Autodesk Fusion 360 part; units mm, degrees
(part 2 of 2)
sketch "Skizze22" plane through (0, -5, 0) normal (0, -1, 0) x (1, 0, 0)
  line L0 (186.6306, 4.2829) -> (187.8211, 23.7465)
  line L1 (187.8211, 23.7465) -> (186.6306, 24.2829)
  line L2 (186.6306, 24.2829) -> (151.6306, 24.2829)
  line L3 (151.6306, 24.2829) -> (151.6306, 40.8836)
  line L4 (-70, 29.3498) -> (-70, 5)
  line L5 (-70, 5) -> (0, 5)
  line L6 (0, 5) -> (0, 4)
  line L7 (0, 4) -> (20, 4)
  line L8 (20, 4) -> (20, 5)
  line L9 (20, 5) -> (149.0505, 5)
  line L10 (87.5, 37.1956) -> (87.5, 52.1956)
  arc A0 (87.5, 52.1956) -> (72.5, 52.1956) centre (80, 52.1956) ccw
  line L11 (72.5, 52.1956) -> (72.5, 37.1956)
  arc A1 (72.5, 37.1956) -> (87.5, 37.1956) centre (80, 37.1956) ccw
  line L12 (80, 37.1956) -> (80, 52.1956) construction
  spline S0 degree 3 poles (14.5724, 48.6404) (30.2605, 50.3322) (46.1682, 51.5352) (61.9632, 52) knots -4.74056 -4.74056 -4.74056 -4.74056 0 0 0 0
  line L13 (151.6306, 4.2829) -> (186.6306, 4.2829)
  arc A2 (151.6306, 4.2829) -> (149.0505, 5) centre (149.0505, 0) ccw
  arc A3 (10, 36.2706) -> (4.2111, 41.2079) centre (5, 36.2706) ccw
  line L14 (4.2111, 41.2079) -> (-70, 29.3498)
  line L15 (20, 43.6831) -> (20, 20)
  line L16 (20, 20) -> (16, 20)
  arc A4 (10, 26) -> (16, 20) centre (16, 26) ccw
  line L17 (10, 26) -> (10, 36.2706)
  line L18 (151.6306, 40.8836) -> (20, 43.6831)
  dimension "d583" = 15
  dimension "d584" = 7.5
  dimension "d710" = 60
  constraint tangent L10 A0
  constraint tangent A0 L11
  constraint parallel L10 L11
  constraint tangent L11 A1
  constraint tangent L10 A1
  constraint vertical L12
  constraint coincident A0.centre S0
  measures "d583" distance of A1.centre A0.centre
  measures "d584" radius of A0
  measures "d710" distance of L12 L15
extrude "Extrusion27" cut sketch "Skizze22" against normal up to surface (6 mm away) contours L10 A0 L11 L18 | L10 L11 A1 L18
sketch "Skizze23" plane through (0, 0, 0) normal (0, 1, 0) x (-1, 0, 0)
  line L0 (0, 4) -> (0, -4)
  line L1 (0, -4) -> (-20, -4)
  line L2 (-20, -4) -> (-20, 4)
  line L3 (-20, 4) -> (0, 4)
  spline S0 degree 5 poles (70.2103, -10.2279) (69.0236, -10.2308) (66.4185, -10.2352) (62.6894, -10.2341) (58.249, -10.2174) (53.3951, -10.1754) (48.6251, -10.1176) (43.5655, -10.0567) (37.7033, -10.0032) (30.7308, -9.9668) (22.6822, -9.9539) (13.8331, -9.9683) (4.596, -10.0103) (-4.5823, -10.0771) (-13.3225, -10.1622) (-21.4171, -10.255) (-28.9285, -10.3413) (-36.0923, -10.4029) (-43.2306, -10.4191) (-50.6596, -10.3663) (-58.6056, -10.2202) (-67.1032, -9.953) (-75.9974, -9.5463) (-85.0071, -8.9937) (-93.7205, -8.3341) (-101.7213, -7.6113) (-108.4203, -7.0066) (-113.6005, -6.5493) (-118.0962, -5.6856) (-122.6878, -3.918) (-127.2425, -1.2895) (-130.2176, 1.0414) (-131.5892, 2.6111) (-132.0631, 3.5029) (-132.1892, 3.8472) knots -0.850912 -0.850912 -0.850912 -0.850912 -0.850912 -0.850912 -0.828571 -0.8 -0.771429 -0.742857 -0.714286 -0.685714 -0.657143 -0.628571 -0.6 -0.571429 -0.542857 -0.514286 -0.485714 -0.457143 -0.428571 -0.4 -0.371429 -0.342857 -0.314286 -0.285714 -0.257143 -0.228571 -0.2 -0.171429 -0.142857 -0.114286 -0.085714 -0.057143 -0.028571 -0.009156 -0.009156 -0.009156 -0.009156 -0.009156 -0.009156
  line L4 (70.2103, -10.2279) -> (70.2103, 1.196)
  spline S1 degree 3 poles (-132.1892, 3.8472) (-132.2839, 4.1058) (-132.3386, 4.3762) (-132.3386, 4.6214) (-132.3386, 5.5356) (-131.713, 6.5125) (-130.5553, 7.509) (-129.4361, 8.4725) (-127.8269, 9.4501) (-125.9058, 10.3673) (-124.0485, 11.2542) (-121.9054, 12.0815) (-119.6316, 12.8016) (-117.4332, 13.4978) (-115.1126, 14.0945) (-112.7619, 14.5861) (-110.4892, 15.0615) (-108.1879, 15.4397) (-105.9044, 15.7378) (-101.5423, 16.3073) (-97.2631, 16.5879) (-93.1078, 16.7673) (-89.2251, 16.9348) (-85.4384, 17.0206) (-81.6004, 17.0826) (-78.0143, 17.1405) (-74.3739, 17.1725) (-70.5512, 17.1644) (-66.9793, 17.1567) (-63.2425, 17.1108) (-59.3309, 17.012) (-55.676, 16.9197) (-51.8726, 16.7815) (-48.0153, 16.6027) (-44.4111, 16.4356) (-40.7643, 16.2337) (-37.1785, 16.0077) (-33.828, 15.7966) (-30.5333, 15.5647) (-27.3568, 15.3189) (-24.3888, 15.0892) (-21.5254, 14.8475) (-18.7699, 14.5932) (-16.1951, 14.3556) (-13.7132, 14.1067) (-11.2856, 13.8408) (-9.0173, 13.5922) (-6.7952, 13.3285) (-4.571, 13.0433) (-0.4647, 12.5168) (3.6588, 11.9145) (8.0916, 11.2103) (11.9497, 10.5975) (16.0436, 9.9077) (20.4372, 9.155) (24.2612, 8.4998) (28.3084, 7.7979) (32.559, 7.0715) (36.2585, 6.4393) (40.1104, 5.7889) (44.0828, 5.1377) (50.9142, 4.0179) (58.0958, 2.8987) (65.4594, 1.8553) (67.0348, 1.632) (68.6189, 1.4121) (70.2103, 1.196) knots 0 0 0 0 0.00882694 0.00882694 0.00882694 0.04173953 0.04173953 0.04173953 0.07355923 0.07355923 0.07355923 0.10432234 0.10432234 0.10432234 0.13406394 0.13406394 0.13406394 0.16281794 0.16281794 0.16281794 0.21774546 0.21774546 0.21774546 0.26906918 0.26906918 0.26906918 0.31702555 0.31702555 0.31702555 0.3618355 0.3618355 0.3618355 0.40370548 0.40370548 0.40370548 0.44282836 0.44282836 0.44282836 0.47938439 0.47938439 0.47938439 0.51354198 0.51354198 0.51354198 0.54545849 0.54545849 0.54545849 0.57528096 0.57528096 0.57528096 0.63034008 0.63034008 0.63034008 0.67826152 0.67826152 0.67826152 0.7199706 0.7199706 0.7199706 0.75627265 0.75627265 0.75627265 0.81870207 0.81870207 0.81870207 0.8320585 0.8320585 0.8320585 0.8320585
  circle A0 centre (34.5409, -4.2358) radius 5
  circle A1 centre (-29.403, -4.3055) radius 5
  arc A2 (39.5409, -4.2303) -> (29.5409, -4.2412) centre (34.5409, -4.2358) ccw
  arc A3 (39.5409, -4.2303) -> (29.5409, -4.2412) centre (34.5409, -4.2358) ccw
  arc A4 (-24.403, -4.3055) -> (-34.403, -4.3055) centre (-29.403, -4.3055) ccw
  arc A5 (-24.403, -4.3055) -> (-34.403, -4.3055) centre (-29.403, -4.3055) ccw
  dimension "d663" = 10
  constraint equal A0 A1
  constraint coincident A1.centre A4.centre
  constraint coincident A0.centre A2.centre
  measures "d663" diameter of A0
extrude "Extrusion29" cut sketch "Skizze23" against normal blind 40 contours A0 A2 A3 | A1 A4 A5
equation "d148 = d143"
equation "d254 = d253 + 0.5 mm"
equation "d306 = d305"
equation "d355 = 87.0 deg - 90 deg"
equation "d716 = d253"
